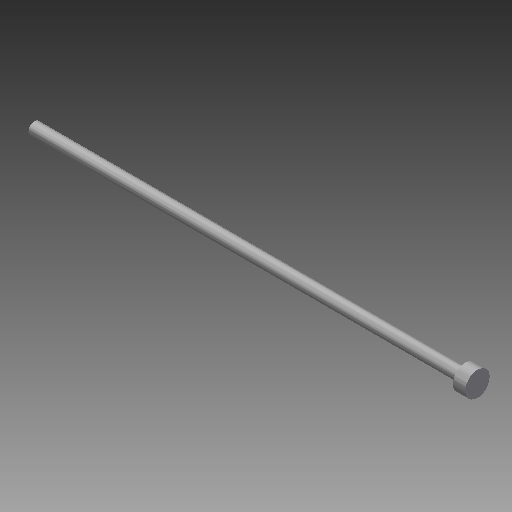
# Autodesk Inventor part: Shaft
Saved by Autodesk Inventor 2017 (Build 210142000, 142)
## iProperties
Created: 2017-11-23
Part Number: Shaft
Material: Steel
Document SubType Name: Modeling
Designer: Biscuit
Density: 1 g/cm^3
Appearance: Steel
CustomPartVersion: 1
Author: Biscuit
Autodesk Inventor part; units mm, degrees
ref_plane "Start Plane" through (0, 0, 0) normal (1, 0, 0) x (0, 1, 0)
ref_plane "XZ Plane" through (0, 0, 0) normal (0, 1, 0) x (-1, 0, 0)
ref_plane "XY Plane" through (0, 0, 0) normal (0, 0, 1) x (1, 0, 0)
sketch "Main Sketch" plane through (0, 0, 0) normal (0, 0, 1) x (1, 0, 0)
  line L0 (0, 0) -> (72, 0)
  line L1 (0, 0) -> (0, 1)
  line L2 (0, 1) -> (70, 1)
  line L3 (70, 1) -> (70, 2)
  line L4 (72, 2) -> (72, 0)
  line L5 (70, 2) -> (72, 2)
  dimension "d3" = 2
  dimension "d4" = 4
  constraints: 12 end point, 4 horizontal, 3 vertical
  measures "d3" diameter of L2 L0
  measures "d4" diameter of L5 L0
revolve "Revolution1" add sketch "Main Sketch" angle 360 about axis through (0, 0, 0) along (1, 0, 0)
body "Solid1"
